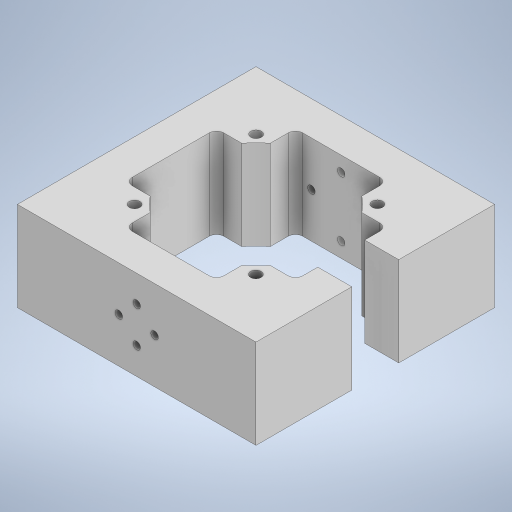
# Autodesk Inventor part: FrontPlateV2
Saved by Autodesk Inventor 2024 (Build 280153000, 153)
## iProperties
Created: 2024-02-08
Part Number: FrontPlateV2
Material: Generic
Document SubType Name: Modeling
Designer: yusuf
Density: 1 g/cm^3
Appearance: Default
Author: yusuf
Autodesk Inventor part; units mm, degrees
ref_plane "YZ Plane" through (0, 0, 0) normal (1, 0, 0) x (0, 1, 0)
ref_plane "XZ Plane" through (0, 0, 0) normal (0, 1, 0) x (-1, 0, 0)
ref_plane "XY Plane" through (0, 0, 0) normal (0, 0, 1) x (1, 0, 0)
sketch "Sketch15" plane through (0, 0, 0) normal (0, 1, 0) x (-1, 0, 0)
  line L0 (0, 0) -> (203.2, 0)
  line L1 (203.2, 0) -> (203.2, -203.2)
  line L2 (203.2, -203.2) -> (0, -203.2)
  line L3 (0, -203.2) -> (0, 0)
  dimension "d149" = 203.2
  dimension "d150" = 203.2
  constraints: 8 end point, 2 parallel, 1 horizontal, 1 perpendicular
  measures "d149" distance of L0.end L1.end
  measures "d150" distance of L1.end L2.end
extrude "Extrusion15" add sketch "Sketch15" along normal blind 76.2
sketch "Sketch16" plane through (0, 76.2, 0) normal (0, 1, 0) x (1, 0, 0)
  line L0 (-166.6, 166.6) -> (-36.6, 166.6)
  line L1 (-36.6, 166.6) -> (-36.6, 36.6)
  line L2 (-36.6, 36.6) -> (-166.6, 36.6)
  line L3 (-166.6, 36.6) -> (-166.6, 166.6)
  line L4 (0, 0) -> (0, 203.2) projected
  dimension "d153" = 130
  dimension "d154" = 130
  dimension "d155" = 36.6
  dimension "d156" = 36.6
  constraints: 8 end point, 2 parallel, 1 horizontal, 1 perpendicular
  measures "d153" distance of L1.end L2.end
  measures "d154" distance of L0.end L1.end
  measures "d155" horizontal distance of L4.start L1.end
  measures "d156" distance between parallel lines of L4 L1
extrude "Extrusion16" cut sketch "Sketch16" against normal through all
sketch "Sketch17" plane through (-203.2, 0, 0) normal (0, 0, 1) x (1, 0, 0)
  line L0 (203.2, 0) -> (0, 0) projected
  line L1 (0, 0) -> (0, 38.1)
  line L2 (0, 38.1) -> (101.6, 38.1)
  circle A0 centre (116.84, 38.1) radius 3.175
  circle A1 centre (101.6, 53.34) radius 3.175
  circle A2 centre (86.36, 38.1) radius 3.175
  circle A3 centre (101.6, 22.86) radius 3.175
  dimension "d159" = 101.6
  dimension "d160" = 38.1
  dimension "d161" = 6.35
  dimension "d162" = 15.24
  dimension "d163" = 0
  dimension "d166" = 360
  constraints: 4 centre point, 4 end point, 1 perpendicular, 1 vertical, 9 other
  measures "d159" distance of L1.end L2.end
  measures "d160" distance of L0.end L1.end
  measures "d161" diameter of A0
  measures "d162" distance of L2.end A0.centre
  measures "d163" vertical distance of A0.centre L2.end
extrude "Extrusion17" cut sketch "Sketch17" against normal blind 101.6
sketch "Sketch19" plane through (0, 76.2, 0) normal (0, 1, 0) x (1, 0, 0)
  line L0 (-36.6, 36.6) -> (-36.6, 166.6) projected
  line L1 (-36.6, 121.6) -> (0.103, 121.6)
  line L2 (0.103, 121.6) -> (0.103, 81.6)
  line L3 (0.103, 81.6) -> (-36.6, 81.6)
  line L4 (-36.6, 81.6) -> (-36.6, 121.6)
  line L5 (-166.6, 166.6) -> (-36.6, 166.6) projected
  point P0 (0, 0)
  dimension "d170" = 40
  dimension "d171" = 45
  dimension "d172" = 36.703
  constraints: 8 end point, 2 parallel, 1 horizontal, 1 perpendicular, 1 point on line
  measures "d170" distance of L1.end L2.end
  measures "d171" distance between parallel lines of L5 L1
  measures "d172" distance between parallel lines of L0 L2
sketch "Sketch22" plane through (0, 76.2, 0) normal (0, 1, 0) x (1, 0, 0)
  line L0 (-166.6, 36.6) -> (-166.6, 62.6)
  line L1 (-166.6, 36.6) -> (-140.6, 36.6)
  line L2 (-140.6, 36.6) -> (-140.6, 50.487)
  line L3 (-166.6, 62.6) -> (-152.713, 62.6)
  arc A0 (-152.713, 62.6) -> (-140.6, 50.487) centre (-100.3536, 102.8464) ccw
  circle A1 centre (-153.25, 49.835) radius 4.4958
  line L4 (-166.6, 166.6) -> (-166.6, 140.6)
  line L5 (-166.6, 166.6) -> (-140.6, 166.6)
  line L6 (-166.6, 140.6) -> (-152.713, 140.6)
  line L7 (-140.6, 166.6) -> (-140.6, 152.713)
  arc A2 (-140.6, 152.713) -> (-152.713, 140.6) centre (-100.3536, 100.3536) ccw
  circle A3 centre (-153.25, 153.365) radius 4.4958
  line L8 (-101.6, 36.6) -> (-101.6, 166.6)
  line L9 (-166.6, 166.6) -> (-140.6, 166.6)
  line L10 (-166.6, 140.6) -> (-166.6, 166.6)
  line L11 (-166.6, 36.6) -> (-140.6, 36.6)
  line L12 (-166.6, 166.6) -> (-166.6, 140.6)
  line L13 (-36.6, 36.6) -> (-36.6, 62.6)
  line L14 (-36.6, 36.6) -> (-62.6, 36.6)
  line L15 (-62.6, 36.6) -> (-62.6, 50.487)
  line L16 (-36.6, 62.6) -> (-50.487, 62.6)
  arc A4 (-62.6, 50.487) -> (-50.487, 62.6) centre (-102.8464, 102.8464) ccw
  circle A5 centre (-49.95, 49.835) radius 4.4958
  line L17 (-36.6, 166.6) -> (-36.6, 140.6)
  line L18 (-36.6, 166.6) -> (-62.6, 166.6)
  line L19 (-36.6, 140.6) -> (-50.487, 140.6)
  line L20 (-62.6, 166.6) -> (-62.6, 152.713)
  arc A6 (-50.487, 140.6) -> (-62.6, 152.713) centre (-102.8464, 100.3536) ccw
  circle A7 centre (-49.95, 153.365) radius 4.4958
  point P0 (0, 0)
  dimension "d191" = 26
  dimension "d206" = 13.887
  dimension "d207" = 13.887
  dimension "d208" = 66.04
  dimension "d210" = 13.35
  dimension "d214" = 8.9916
  dimension "d217" = 12.765
  dimension "d218" = 26
  dimension "d219" = 26
  dimension "d220" = 13.887
  dimension "d221" = 13.887
  dimension "d222" = 66.04
  dimension "d223" = 8.9916
  dimension "d224" = 12.765
  dimension "d225" = 13.35
  dimension "d232" = 90
  dimension "d233" = 26
  dimension "d234" = 65
  dimension "d235" = 130
  dimension "d236" = 0
  constraints: 42 end point, 14 symmetric about line, 8 centre point, 8 point on circle, 3 horizontal, 3 parallel, 2 vertical, 1 collinear, 4 other
  measures "d191" distance of L0.start L0.end
  measures "d206" distance of L1.end L2.end
  measures "d207" distance of L0.end L3.end
  measures "d208" radius of A0
  measures "d210" distance from line of L0 A1.centre
  measures "d214" diameter of A1
  measures "d217" vertical distance of L0.end A1.centre
  measures "d218" distance of L4.start L5.end
  measures "d219" distance of L4.start L4.end
  measures "d220" distance of L4.end L6.end
  measures "d221" distance of L5.end L7.end
  measures "d222" radius of A2
  measures "d223" diameter of A3
  measures "d224" vertical distance of L4.end A3.centre
  measures "d225" horizontal distance of L4.end A3.centre
  measures "d232" angle of L13 L14
  measures "d233" distance between parallel lines of L15 L17
  measures "d234" distance between parallel lines of L17 L8
  measures "d235" distance from line of L8.end L14
  measures "d236" distance from line of L8.start L14
sketch "Sketch23" plane through (0, 0, -203.2) normal (0, 0, -1) x (-1, 0, 0)
  line L0 (0, 0) -> (0, 38.1)
  circle A0 centre (127, 38.1) radius 3.175
  line L1 (0, 38.1) -> (101.6, 38.1)
  circle A1 centre (101.6, 63.5) radius 3.175
  circle A2 centre (76.2, 38.1) radius 3.175
  circle A3 centre (101.6, 12.7) radius 3.175
  dimension "d180" = 101.6
  dimension "d181" = 38.1
  dimension "d182" = 25.4
  dimension "d183" = 0
  dimension "d184" = 6.35
  dimension "d187" = 360
  constraints: 4 centre point, 4 end point, 1 horizontal, 1 vertical, 9 other
  measures "d180" distance of L0.end L1.end
  measures "d181" distance of L0.start L0.end
  measures "d182" distance of L1.end A0.centre
  measures "d183" vertical distance of L1.end A0.centre
  measures "d184" diameter of A0
extrude "Extrusion20" cut sketch "Sketch23" against normal blind 101.6
extrude "Extrusion28" add sketch "Sketch22" against normal blind 76.2
sketch "Sketch26" plane through (0, 76.2, 0) normal (0, 1, 0) x (1, 0, 0)
  line L0 (-62.6, 166.6) -> (-140.6, 166.6)
  line L1 (-140.6, 166.6) -> (-140.6, 174.22)
  line L2 (-140.6, 174.22) -> (-62.6, 174.22)
  line L3 (-62.6, 174.22) -> (-62.6, 166.6)
  line L4 (-140.6, 152.713) -> (-140.6, 166.6) projected
  line L5 (-140.6, 36.6) -> (-140.6, 50.487) projected
  line L6 (-140.6, 36.6) -> (-62.6, 36.6)
  line L7 (-62.6, 36.6) -> (-62.6, 28.98)
  line L8 (-62.6, 28.98) -> (-140.6, 28.98)
  line L9 (-140.6, 28.98) -> (-140.6, 36.6)
  line L10 (-62.6, 50.487) -> (-62.6, 36.6) projected
  point P0 (0, 0)
  dimension "d242" = 0
  dimension "d243" = 7.62
  dimension "d244" = 0
  dimension "d245" = 7.62
  constraints: 16 end point, 4 parallel, 2 horizontal, 2 perpendicular
  measures "d242" distance between parallel lines of L4 L1
  measures "d243" distance between parallel lines of L0 L2
  measures "d244" distance between parallel lines of L10 L7
  measures "d245" distance between parallel lines of L6 L8
extrude "Extrusion29" cut sketch "Sketch26" against normal through all
sketch "Sketch28" plane through (0, 76.2, 0) normal (0, 1, 0) x (1, 0, 0)
  line L0 (-166.6, 140.6) -> (-166.6, 62.6) projected
  line L1 (-166.6, 140.6) -> (-174.22, 140.6)
  line L2 (-174.22, 140.6) -> (-174.22, 62.6)
  line L3 (-174.22, 62.6) -> (-166.6, 62.6)
  line L4 (-166.6, 62.6) -> (-166.6, 140.6)
  line L5 (-152.713, 62.6) -> (-166.6, 62.6) projected
  line L6 (-36.6, 62.6) -> (-36.6, 140.6) projected
  line L7 (-36.6, 62.6) -> (-28.98, 62.6)
  line L8 (-28.98, 62.6) -> (-28.98, 140.6)
  line L9 (-28.98, 140.6) -> (-36.6, 140.6)
  line L10 (-36.6, 140.6) -> (-36.6, 62.6)
  line L11 (-50.487, 140.6) -> (-36.6, 140.6) projected
  point P0 (0, 0)
  point P1 (-170.41, 62.6)
  dimension "d253" = 0
  dimension "d254" = 7.62
  dimension "d255" = 0
  dimension "d256" = 7.62
  constraints: 16 end point, 4 parallel, 2 horizontal, 2 perpendicular, 1 midpoint
  measures "d253" distance from line of L5 point (-170.41, 62.6)
  measures "d254" distance between parallel lines of L0 L2
  measures "d255" distance between parallel lines of L11 L9
  measures "d256" distance between parallel lines of L6 L8
extrude "Extrusion30" cut sketch "Sketch28" against normal through all
fillet "Fillet9" radius 6.35 8 edges at (-140.6, 38.1, -174.22) (-62.6, 38.1, -174.22) (-28.98, 38.1, -140.6) (-28.98, 38.1, -62.6) (-62.6, 38.1, -28.98) (-140.6, 38.1, -28.98) (-174.22, 38.1, -62.6) (-174.22, 38.1, -140.6)
extrude "Extrusion31" cut sketch "Sketch19" against normal through all
body "Solid2"
